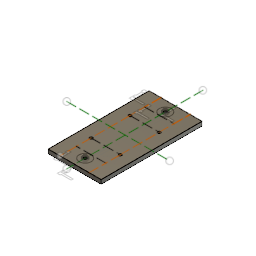
Plunging_solenoid_holderV1 (Autodesk Fusion 360 design; units mm, degrees)
Autodesk Fusion 360 part; units mm, degrees
sketch "Sketch1" plane through (0, 0, 0) normal (0, 1, 0) x (1, 0, 0)
  line L0 (-27.26, -52) -> (-27.26, 52)
  line L1 (-27.26, 52) -> (27.26, 52)
  line L2 (27.26, 52) -> (27.26, -52)
  line L3 (0, 80) -> (0, -60) construction
  line L4 (-60, 0) -> (45.848, 0) construction
  line L5 (-15, 52) -> (-15, 35.15) construction
  line L6 (-15, 35.15) -> (15, 35.15) construction
  line L7 (15, 35.15) -> (15, 52) construction
  circle A0 centre (0, 41.325) radius 6.175
  line L8 (-15, 52) -> (-15, 20) construction
  line L9 (-15, 20) -> (15, 20) construction
  line L10 (15, 20) -> (15, 52) construction
  line L11 (-15, 20) -> (-15, -20) construction
  line L12 (-15, -20) -> (15, -20) construction
  line L13 (15, -20) -> (15, 20) construction
  line L14 (27.26, -52) -> (-27.26, -52)
  line L15 (15, -52) -> (15, -35) construction
  line L16 (15, -35) -> (-15, -35) construction
  line L17 (-15, -35) -> (-15, -52) construction
  line L18 (-15, -20) -> (-15, -35) construction
  line L19 (15, -20) -> (15, -35) construction
  circle A1 centre (0, -41.175) radius 6.175
  dimension "d2" = 54.52
  dimension "d6" = 16.85
  dimension "d7" = 12.35
  dimension "d9" = 32
  dimension "d10" = 40
  dimension "d12" = 104
  dimension "d16" = 17
  dimension "d17" = 12.35
  measures "d7" diameter of A0
  measures "d17" diameter of A1
extrude "Extrude1" add sketch "Sketch1" against normal blind 4.3 contours L0 L1 L2 L14 | A0 | A1
sketch "Sketch2" plane through (0, 0, 0) normal (0, 1, 0) x (1, 0, 0)
  circle A0 centre (-15, -20) radius 1.5
  circle A1 centre (15, -20) radius 1.5
  circle A2 centre (-15, 20) radius 1.5
  circle A3 centre (15, 20) radius 1.5
  circle A4 centre (0, 41.325) radius 1.5
  circle A5 centre (0, -41.175) radius 1.5
  dimension "d20" = 3
  dimension "d21" = 3
  dimension "d22" = 3
  dimension "d23" = 3
  dimension "d24" = 3
  dimension "d25" = 3
  measures "d20" diameter of A0
  measures "d21" diameter of A1
  measures "d22" diameter of A2
  measures "d23" diameter of A3
  measures "d24" diameter of A4
  measures "d25" diameter of A5
extrude "Extrude2" cut sketch "Sketch2" against normal up to surface (4.3 mm away)
